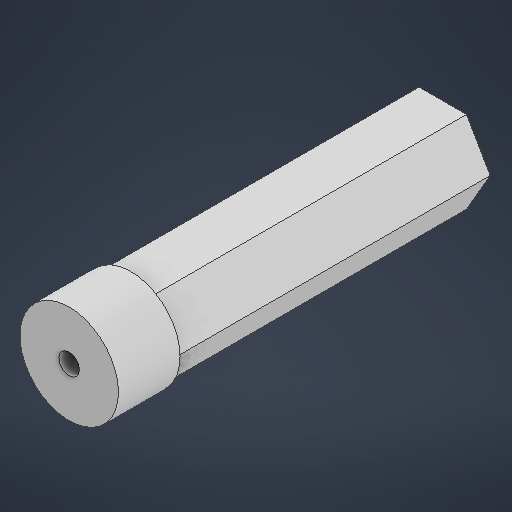
# Autodesk Inventor part: Shaft
Saved by Autodesk Inventor 2026 (Build 300175050, 175E)
## iProperties
Created: 2025-11-03
Part Number: Shaft
Material: Generic
Document SubType Name: Modeling
Designer: randy
Density: 1 g/cm^3
Appearance: Default
Author: randy
Autodesk Inventor part; units mm, degrees
ref_plane "YZ Plane" through (0, 0, 0) normal (1, 0, 0) x (0, 1, 0)
ref_plane "XZ Plane" through (0, 0, 0) normal (0, 1, 0) x (-1, 0, 0)
ref_plane "XY Plane" through (0, 0, 0) normal (0, 0, 1) x (1, 0, 0)
sketch "Sketch1" plane through (0, 0, 0) normal (0, 0, 1) x (1, 0, 0)
  line L0 (-7.3323, 0) -> (-3.6662, 6.35)
  line L1 (-3.6662, 6.35) -> (3.6662, 6.35)
  line L2 (3.6662, 6.35) -> (7.3323, 0)
  line L3 (7.3323, 0) -> (3.6662, -6.35)
  line L4 (3.6662, -6.35) -> (-3.6662, -6.35)
  line L5 (-3.6662, -6.35) -> (-7.3323, 0)
  circle A0 centre (0, 0) radius 1.5923
  dimension "d0" = 12.7
  constraints: 12 end point, 2 coincident, 1 centre point, 1 horizontal, 13 other
  measures "d0" distance between parallel lines of L4 L1
extrude "Extrusion1" add sketch "Sketch1" along normal mid plane 48.26
sketch "Sketch2" plane through (0, 0, 24.13) normal (0, 0, 1) x (1, 0, 0)
  line L0 (3.6662, 6.35) -> (-3.6662, 6.35) projected
  line L1 (-3.6662, -6.35) -> (3.6662, -6.35) projected
  line L2 (3.6662, -6.35) -> (7.3323, 0) projected
  line L3 (7.3323, 0) -> (3.6662, 6.35) projected
  line L4 (3.6662, 6.35) -> (-3.6662, 6.35) projected
  line L5 (-3.6662, 6.35) -> (-7.3323, 0) projected
  line L6 (-7.3323, 0) -> (-3.6662, -6.35) projected
  circle A0 centre (0, 0) radius 1.5923 projected
  circle A1 centre (0, 0) radius 7.62
  dimension "d5" = 15.24
  constraints: 1 centre point, 1 coincident
  measures "d5" diameter of A1
extrude "Extrusion2" add sketch "Sketch2" along normal blind 9.525 contours L3 L2 L1 L6 L5 L0 | A1
body "Solid1"
